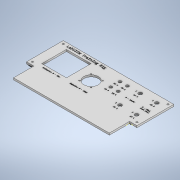
# Autodesk Inventor part: Labview Training Faceplate
Saved by Autodesk Inventor 2022 (Build 260153000, 153)
## iProperties
Created: 2022-07-29
Part Number: Labview Training Faceplate
Material: Generic
Document SubType Name: Modeling
Designer: dheard
Density: 1 g/cm^3
Appearance: Default
Author: dheard
Autodesk Inventor part; units mm, degrees
(part 1 of 3)
ref_plane "YZ Plane" through (0, 0, 0) normal (1, 0, 0) x (0, 1, 0)
ref_plane "XZ Plane" through (0, 0, 0) normal (0, 1, 0) x (-1, 0, 0)
ref_plane "XY Plane" through (0, 0, 0) normal (0, 0, 1) x (1, 0, 0)
sketch "Sketch1" plane through (0, 0, 0) normal (0, 1, 0) x (-1, 0, 0)
  line L0 (150, -50) -> (-150, -50)
  line L1 (-150, -50) -> (-150, 50)
  line L2 (150, 50) -> (150, -50)
  line L3 (-130, 50) -> (-130, 105)
  line L4 (-130, 105) -> (130, 105)
  line L5 (130, 105) -> (130, 50)
  line L6 (-150, 50) -> (-130, 50)
  line L7 (130, 50) -> (150, 50)
  point P0 (0, 0)
  dimension "d0" = 100
  dimension "d1" = 55
  dimension "d2" = 300
  dimension "d3" = 20
  dimension "d4" = 20
  dimension "d5" = 150
  dimension "d6" = 50
  constraints: 16 end point, 4 parallel, 2 horizontal alignment, 1 horizontal, 1 perpendicular
  measures "d0" distance between parallel lines of L7 L0
  measures "d1" distance between parallel lines of L4 L7
  measures "d2" distance between parallel lines of L1 L2
  measures "d3" distance between parallel lines of L5 L2
  measures "d4" distance between parallel lines of L1 L3
  measures "d5" distance from line of point (0, 0) L1
  measures "d6" distance from line of point (0, 0) L0
extrude "Extrusion1" add sketch "Sketch1" along normal blind 5
sketch "Sketch3" plane through (0, 5, 0) normal (0, 1, 0) x (1, 0, 0)
  line L0 (-125, 33.5) -> (-58, 33.5)
  line L1 (-58, 33.5) -> (-58, -33.5)
  line L2 (-58, -33.5) -> (-125, -33.5)
  line L3 (-125, -33.5) -> (-125, 33.5)
  line L4 (150, 50) -> (-150, 50) projected
  line L5 (-150, 50) -> (-150, -50) projected
  circle A0 centre (-18, -6.5) radius 19.5
  line L6 (-34, 9.5) -> (-2, 9.5) construction
  line L7 (-2, 9.5) -> (-2, -22.5) construction
  line L8 (-2, -22.5) -> (-34, -22.5) construction
  line L9 (-34, -22.5) -> (-34, 9.5) construction
  circle A1 centre (-34, 9.5) radius 1.5
  circle A2 centre (-2, -22.5) radius 1.5
  circle A3 centre (-34, -22.5) radius 1.5
  circle A4 centre (-2, 9.5) radius 1.5
  circle A5 centre (79, -25) radius 4.75
  circle A6 centre (79, 30) radius 4.75
  circle A7 centre (124, -25) radius 4.75
  circle A8 centre (124, 30) radius 4.75
  circle A9 centre (24, 5) radius 4
  circle A10 centre (44, 5) radius 4
  circle A11 centre (44, 30) radius 4
  circle A12 centre (24, 30) radius 4
  line L10 (68, 31.3) -> (68, 28.7) construction
  line L11 (68.65, 31.3) -> (68.65, 28.7)
  line L12 (67.35, 28.7) -> (67.35, 31.3)
  arc A13 (68.65, 31.3) -> (67.35, 31.3) centre (68, 31.3) ccw
  arc A14 (67.35, 28.7) -> (68.65, 28.7) centre (68, 28.7) ccw
  line L13 (68, -23.7) -> (68, -26.3) construction
  line L14 (68.65, -23.7) -> (68.65, -26.3)
  line L15 (67.35, -26.3) -> (67.35, -23.7)
  arc A15 (68.65, -23.7) -> (67.35, -23.7) centre (68, -23.7) ccw
  arc A16 (67.35, -26.3) -> (68.65, -26.3) centre (68, -26.3) ccw
  line L16 (112.35, -26.3) -> (112.35, -23.7)
  line L17 (113, -23.7) -> (113, -26.3) construction
  line L18 (113.65, -23.7) -> (113.65, -26.3)
  arc A17 (113.65, -23.7) -> (112.35, -23.7) centre (113, -23.7) ccw
  arc A18 (112.35, -26.3) -> (113.65, -26.3) centre (113, -26.3) ccw
  line L19 (112.35, 28.7) -> (112.35, 31.3)
  line L20 (113, 31.3) -> (113, 28.7) construction
  line L21 (113.65, 31.3) -> (113.65, 28.7)
  arc A19 (113.65, 31.3) -> (112.35, 31.3) centre (113, 31.3) ccw
  arc A20 (112.35, 28.7) -> (113.65, 28.7) centre (113, 28.7) ccw
  line L22 (-150, -50) -> (-130, -50) projected
  point P0 (68, 30)
  point P1 (68, -25)
  point P2 (113, -25)
  point P3 (113, 30)
  dimension "d11" = 67
  dimension "d12" = 67
  dimension "d13" = 16.5
  dimension "d15" = 25
  dimension "d16" = 39
  dimension "d17" = 40
  dimension "d18" = 40
  dimension "d19" = 32
  dimension "d20" = 32
  dimension "d23" = 16
  dimension "d24" = 16
  dimension "d25" = 3
  dimension "d26" = 3
  dimension "d27" = 3
  dimension "d28" = 3
  dimension "d29" = 9.5
  dimension "d30" = 45
  dimension "d31" = 55
  dimension "d32" = 20
  dimension "d34" = 8
  dimension "d36" = 20
  dimension "d37" = 25
  dimension "d38" = 20
  dimension "d39" = 42
  dimension "d40" = 35
  dimension "d41" = 11
  dimension "d42" = 2.6
  dimension "d43" = 1.3
  dimension "d44" = 2.6
  dimension "d45" = 1.3
  dimension "d46" = 2.6
  dimension "d47" = 1.3
  dimension "d48" = 2.6
  dimension "d49" = 1.3
  dimension "d50" = 11
  dimension "d65" = 16.5
  constraints: 48 end point, 21 centre point, 16 point on circle, 16 tangent, 8 horizontal alignment, 8 parallel, 6 equal radius, 6 vertical alignment, 4 coincident, 4 midpoint, 4 vertical, 2 horizontal, 2 perpendicular
  measures "d11" distance between parallel lines of L1 L3
  measures "d12" distance between parallel lines of L2 L0
  measures "d13" distance between parallel lines of L4 L0
  measures "d15" distance between parallel lines of L5 L3
  measures "d16" diameter of A0
  measures "d17" distance from line of L0 A0.centre
  measures "d18" distance from line of A0.centre L1
  measures "d19" distance between parallel lines of L7 L9
  measures "d20" distance between parallel lines of L6 L8
  measures "d23" distance from line of A0.centre L6
  measures "d24" distance from line of A0.centre L9
  measures "d25" diameter of A1
  measures "d26" diameter of A4
  measures "d27" diameter of A2
  measures "d28" diameter of A3
  measures "d29" diameter of A5
  measures "d30" distance of A8.centre A6.centre
  measures "d31" distance of A7.centre A8.centre
  measures "d32" distance from line of L4 A6.centre
  measures "d34" diameter of A9
  measures "d36" distance of A10.centre A9.centre
  measures "d37" distance of A10.centre A11.centre
  measures "d38" distance from line of L4 A12.centre
  measures "d39" horizontal distance of A0.centre A12.centre
  measures "d40" distance of A11.centre A6.centre
  measures "d41" distance of A6.centre point (68, 30)
  measures "d42" distance of L10.start L10.end
  measures "d43" distance between parallel lines of L11 L12
  measures "d44" distance of L13.start L13.end
  measures "d45" distance between parallel lines of L14 L15
  measures "d46" distance of L17.start L17.end
  measures "d47" distance between parallel lines of L18 L16
  measures "d48" distance of L20.start L20.end
  measures "d49" distance between parallel lines of L21 L19
  measures "d50" distance of A8.centre point (113, 30)
  measures "d65" distance between parallel lines of L22 L2
extrude "Extrusion2" cut sketch "Sketch3" against normal through all
sketch "Sketch4" plane through (0, 5, 0) normal (0, 1, 0) x (1, 0, 0)
  circle A0 centre (-142, 42) radius 2.25
  circle A1 centre (142, 42) radius 2.25
  circle A2 centre (-142, -42) radius 2.25
  circle A3 centre (142, -42) radius 2.25
  line L0 (-150, 50) -> (-150, -50) projected
  line L1 (150, 50) -> (-150, 50) projected
  line L2 (-150, -50) -> (-130, -50) projected
  line L3 (150, -50) -> (150, 50) projected
  point P0 (0, 0)
  dimension "d55" = 4.5
  dimension "d58" = 8
  dimension "d59" = 8
  dimension "d60" = 8
  dimension "d62" = 8
  constraints: 4 centre point, 3 equal radius, 2 horizontal alignment, 2 vertical alignment
  measures "d55" diameter of A0
  measures "d58" distance from line of L0 A0.centre
  measures "d59" distance from line of L1 A0.centre
  measures "d60" distance from line of L2 A2.centre
  measures "d62" distance from line of L3 A1.centre
extrude "Extrusion3" cut sketch "Sketch4" against normal blind 10
sketch "Sketch5" plane through (0, 5, 0) normal (0, 1, 0) x (1, 0, 0)
  line L0 (-131.9692, 46) -> (-24.524, 46) construction
  line L1 (-24.524, 46) -> (-24.524, 37.1257) construction
  line L2 (-24.524, 37.1257) -> (-131.9692, 37.1257) construction
  line L3 (-131.9692, 37.1257) -> (-131.9692, 46) construction
  line L4 (-115, -39) -> (-68, -39) construction
  line L5 (-68, -39) -> (-68, -43.7381) construction
  line L6 (-68, -43.7381) -> (-115, -43.7381) construction
  line L7 (-115, -43.7381) -> (-115, -39) construction
  line L8 (-41, -43.9686) -> (-41, -39) construction
  line L9 (-41, -39) -> (5, -39) construction
  line L10 (5, -39) -> (5, -43.9686) construction
  line L11 (5, -43.9686) -> (-41, -43.9686) construction
  line L12 (19, 14.2768) -> (19, 20) construction
  line L13 (19, 20) -> (30.6254, 20) construction
  line L14 (30.6254, 20) -> (30.6254, 14.2768) construction
  line L15 (30.6254, 14.2768) -> (19, 14.2768) construction
  line L16 (39, 14.2768) -> (39, 20) construction
  line L17 (39, 20) -> (50.0529, 20) construction
  line L18 (50.0529, 20) -> (50.0529, 14.2768) construction
  line L19 (50.0529, 14.2768) -> (39, 14.2768) construction
  line L20 (19, -10.7232) -> (19, -5) construction
  line L21 (19, -5) -> (31.5796, -5) construction
  line L22 (31.5796, -5) -> (31.5796, -10.7232) construction
  line L23 (31.5796, -10.7232) -> (19, -10.7232) construction
  line L24 (39, -10.7232) -> (39, -5) construction
  line L25 (39, -5) -> (50.0917, -5) construction
  line L26 (50.0917, -5) -> (50.0917, -10.7232) construction
  line L27 (50.0917, -10.7232) -> (39, -10.7232) construction
  line L28 (68, -2.5818) -> (68, 3) construction
  line L29 (68, 3) -> (94.3213, 3) construction
  line L30 (94.3213, 3) -> (94.3213, -2.5818) construction
  line L31 (94.3213, -2.5818) -> (68, -2.5818) construction
  line L32 (113, -2.5818) -> (113, 3) construction
  line L33 (113, 3) -> (139.3213, 3) construction
  line L34 (139.3213, 3) -> (139.3213, -2.5818) construction
  line L35 (139.3213, -2.5818) -> (113, -2.5818) construction
  line L36 (113, -6.8453) -> (113, -2.353) construction
  line L37 (113, -2.353) -> (137.7599, -2.353) construction
  line L38 (137.7599, -2.353) -> (137.7599, -6.8453) construction
  line L39 (137.7599, -6.8453) -> (113, -6.8453) construction
  line L40 (73, 14.4182) -> (73, 20) construction
  line L41 (73, 20) -> (86.5493, 20) construction
  line L42 (86.5493, 20) -> (86.5493, 14.4182) construction
  line L43 (86.5493, 14.4182) -> (73, 14.4182) construction
  line L44 (73, -40.5818) -> (73, -35) construction
  line L45 (73, -35) -> (86.5493, -35) construction
  line L46 (86.5493, -35) -> (86.5493, -40.5818) construction
  line L47 (86.5493, -40.5818) -> (73, -40.5818) construction
  line L48 (118, 14.4182) -> (118, 20) construction
  line L49 (118, 20) -> (131.5493, 20) construction
  line L50 (131.5493, 20) -> (131.5493, 14.4182) construction
  line L51 (131.5493, 14.4182) -> (118, 14.4182) construction
  line L52 (118, -40.5818) -> (118, -35) construction
  line L53 (118, -35) -> (131.5493, -35) construction
  line L54 (131.5493, -35) -> (131.5493, -40.5818) construction
  line L55 (131.5493, -40.5818) -> (118, -40.5818) construction
  circle A0 centre (24, 30) radius 4 projected
  circle A1 centre (24, 5) radius 4 projected
  circle A2 centre (44, 30) radius 4 projected
  circle A3 centre (79, 30) radius 4.75 projected
  circle A4 centre (124, 30) radius 4.75 projected
  circle A5 centre (79, -25) radius 4.75 projected
  line L56 (-150, -50) -> (-130, -50) projected
  line L57 (-125, -33.5) -> (-125, 33.5) projected
  line L58 (-58, 33.5) -> (-58, -33.5) projected
  circle A6 centre (-18, -6.5) radius 19.5 projected
  line L59 (150, 50) -> (-150, 50) projected
  line L60 (-127.3724, 39.3479) -> (-130.8815, 39.3479)
  line L61 (-130.8815, 39.3479) -> (-130.8815, 45.4479)
  line L62 (-130.8815, 45.4479) -> (-130.0343, 45.4479)
  line L63 (-130.0343, 45.4479) -> (-130.0343, 40.0585)
  line L64 (-130.0343, 40.0585) -> (-127.3724, 40.0585)
  line L65 (-127.3724, 40.0585) -> (-127.3724, 39.3479)
  line L66 (-122.9504, 39.3479) -> (-122.9668, 39.9765)
  spline S0 degree 2 poles (-122.9668, 39.9765) (-123.3494, 39.5994) (-124.142, 39.2659) (-124.5738, 39.2659) knots 0 0 0 1 2 2 2
  spline S1 degree 2 poles (-124.5738, 39.2659) (-124.9783, 39.2659) (-125.5467, 39.4737) (-125.913, 39.8289) (-126.0879, 40.3154) (-126.0879, 40.5996) knots 0 0 0 1 2 3 4 4 4
  spline S2 degree 2 poles (-126.0879, 40.5996) (-126.0879, 41.3047) (-125.0384, 42.1028) (-124.0108, 42.1028) knots 0 0 0 1 2 2 2
  line L67 (-124.0108, 42.1028) -> (-123.0379, 42.1028)
  line L68 (-123.0379, 42.1028) -> (-123.0379, 42.5127)
  spline S3 degree 2 poles (-123.0379, 42.5127) (-123.0379, 42.9281) (-123.5681, 43.431) (-124.1147, 43.431) knots 0 0 0 1 2 2 2
  spline S4 degree 2 poles (-124.1147, 43.431) (-124.5137, 43.431) (-125.2844, 43.2561) (-125.6943, 43.0921) knots 0 0 0 1 2 2 2
  line L69 (-125.6943, 43.0921) -> (-125.6943, 43.8246)
  spline S5 degree 2 poles (-125.6943, 43.8246) (-125.5413, 43.8792) (-125.1641, 43.9885) (-124.7433, 44.0705) (-124.2841, 44.1197) (-124.0545, 44.1197) knots 0 0 0 1 2 3 4 4 4
  spline S6 degree 2 poles (-124.0545, 44.1197) (-123.6282, 44.1197) (-122.945, 43.9339) (-122.4749, 43.5513) (-122.2234, 42.9719) (-122.2234, 42.5783) knots 0 0 0 1 2 3 4 4 4
  line L70 (-122.2234, 42.5783) -> (-122.2234, 39.3479)
  line L71 (-122.2234, 39.3479) -> (-122.9504, 39.3479)
  line L72 (-123.0379, 41.4797) -> (-124.0709, 41.4797)
  spline S7 degree 2 poles (-124.0709, 41.4797) (-124.377, 41.4797) (-124.8143, 41.3594) (-125.0931, 41.1353) (-125.2297, 40.8237) (-125.2297, 40.627) knots 0 0 0 1 2 3 4 4 4
  spline S8 degree 2 poles (-125.2297, 40.627) (-125.2297, 40.4903) (-125.1477, 40.2444) (-124.9564, 40.053) (-124.6613, 39.9437) (-124.4426, 39.9437) knots 0 0 0 1 2 3 4 4 4
  spline S9 degree 2 poles (-124.4426, 39.9437) (-124.1639, 39.9437) (-123.4424, 40.2826) (-123.0379, 40.6488) knots 0 0 0 1 2 2 2
  line L73 (-123.0379, 40.6488) -> (-123.0379, 41.4797)
  spline S10 degree 2 poles (-116.6974, 41.7748) (-116.6974, 41.1954) (-117.0199, 40.2717) (-117.6102, 39.6322) (-118.4629, 39.2933) (-118.9931, 39.2933) knots 0 0 0 1 2 3 4 4 4
  spline S11 degree 2 poles (-118.9931, 39.2933) (-119.4085, 39.2933) (-120.2776, 39.4518) (-120.7039, 39.6267) knots 0 0 0 1 2 2 2
  line L74 (-120.7039, 39.6267) -> (-120.7039, 45.9453)
  line L75 (-120.7039, 45.9453) -> (-119.8895, 45.9453)
  line L76 (-119.8895, 45.9453) -> (-119.8895, 44.1306)
  line L77 (-119.8895, 44.1306) -> (-119.9277, 43.2616)
  spline S12 degree 2 poles (-119.9277, 43.2616) (-119.5779, 43.7316) (-118.7799, 44.1197) (-118.3208, 44.1197) knots 0 0 0 1 2 2 2
  spline S13 degree 2 poles (-118.3208, 44.1197) (-117.9217, 44.1197) (-117.315, 43.7863) (-116.9051, 43.1741) (-116.6974, 42.3105) (-116.6974, 41.7748) knots 0 0 0 1 2 3 4 4 4
  spline S14 degree 2 poles (-117.5282, 41.7366) (-117.5282, 42.1082) (-117.6375, 42.7204) (-117.8671, 43.1632) (-118.2333, 43.4091) (-118.4847, 43.4091) knots 0 0 0 1 2 3 4 4 4
  spline S15 degree 2 poles (-118.4847, 43.4091) (-118.6378, 43.4091) (-118.9548, 43.3108) (-119.2992, 43.0812) (-119.6763, 42.704) (-119.8895, 42.4253) knots 0 0 0 1 2 3 4 4 4
  line L78 (-119.8895, 42.4253) -> (-119.8895, 40.1514)
  spline S16 degree 2 poles (-119.8895, 40.1514) (-119.649, 40.0585) (-119.1571, 39.9492) (-118.9329, 39.9492) knots 0 0 0 1 2 2 2
  spline S17 degree 2 poles (-118.9329, 39.9492) (-118.6542, 39.9492) (-118.1458, 40.1241) (-117.7578, 40.5395) (-117.5282, 41.2282) (-117.5282, 41.7366) knots 0 0 0 1 2 3 4 4 4
  line L79 (-110.9527, 45.4479) -> (-113.0297, 39.3479)
  line L80 (-113.0297, 39.3479) -> (-114.1502, 39.3479)
  line L81 (-114.1502, 39.3479) -> (-116.1726, 45.4479)
  line L82 (-116.1726, 45.4479) -> (-115.238, 45.4479)
  line L83 (-115.238, 45.4479) -> (-113.9207, 41.3375)
  line L84 (-113.9207, 41.3375) -> (-113.5435, 40.1296)
  line L85 (-113.5435, 40.1296) -> (-113.1609, 41.3375)
  line L86 (-113.1609, 41.3375) -> (-111.8436, 45.4479)
  line L87 (-111.8436, 45.4479) -> (-110.9527, 45.4479)
  line L88 (-108.728, 44.7483) -> (-110.1328, 44.7483)
  line L89 (-110.1328, 44.7483) -> (-110.1328, 45.4479)
  line L90 (-110.1328, 45.4479) -> (-106.4815, 45.4479)
  line L91 (-106.4815, 45.4479) -> (-106.4815, 44.7483)
  line L92 (-106.4815, 44.7483) -> (-107.8863, 44.7483)
  line L93 (-107.8863, 44.7483) -> (-107.8863, 40.0585)
  line L94 (-107.8863, 40.0585) -> (-106.4815, 40.0585)
  line L95 (-106.4815, 40.0585) -> (-106.4815, 39.3479)
  line L96 (-106.4815, 39.3479) -> (-110.1328, 39.3479)
  line L97 (-110.1328, 39.3479) -> (-110.1328, 40.0585)
  line L98 (-110.1328, 40.0585) -> (-108.728, 40.0585)
  line L99 (-108.728, 40.0585) -> (-108.728, 44.7483)
  line L100 (-101.267, 39.3479) -> (-104.7379, 39.3479)
  line L101 (-104.7379, 39.3479) -> (-104.7379, 45.4479)
  line L102 (-104.7379, 45.4479) -> (-101.267, 45.4479)
  line L103 (-101.267, 45.4479) -> (-101.267, 44.7483)
  line L104 (-101.267, 44.7483) -> (-103.9071, 44.7483)
  line L105 (-103.9071, 44.7483) -> (-103.9071, 42.8571)
  line L106 (-103.9071, 42.8571) -> (-101.3708, 42.8571)
  line L107 (-101.3708, 42.8571) -> (-101.3708, 42.1574)
  line L108 (-101.3708, 42.1574) -> (-103.9071, 42.1574)
  line L109 (-103.9071, 42.1574) -> (-103.9071, 40.0585)
  line L110 (-103.9071, 40.0585) -> (-101.267, 40.0585)
  line L111 (-101.267, 40.0585) -> (-101.267, 39.3479)
  line L112 (-95.3747, 45.4479) -> (-95.7846, 39.3479)
  line L113 (-95.7846, 39.3479) -> (-96.8614, 39.3479)
  line L114 (-96.8614, 39.3479) -> (-97.6212, 41.5179)
  line L115 (-97.6212, 41.5179) -> (-97.8289, 42.2121)
  line L116 (-97.8289, 42.2121) -> (-98.0476, 41.4633)
  line L117 (-98.0476, 41.4633) -> (-98.7527, 39.3479)
  line L118 (-98.7527, 39.3479) -> (-99.7912, 39.3479)
  line L119 (-99.7912, 39.3479) -> (-100.2121, 45.4479)
  line L120 (-100.2121, 45.4479) -> (-99.4304, 45.4479)
  line L121 (-99.4304, 45.4479) -> (-99.1899, 41.2938)
  line L122 (-99.1899, 41.2938) -> (-99.1189, 40.1569)
  line L123 (-99.1189, 40.1569) -> (-98.8237, 41.1244)
  line L124 (-98.8237, 41.1244) -> (-98.0858, 43.3873)
  line L125 (-98.0858, 43.3873) -> (-97.5119, 43.3873)
  line L126 (-97.5119, 43.3873) -> (-96.6592, 40.9604)
  line L127 (-96.6592, 40.9604) -> (-96.375, 40.1569)
  line L128 (-96.375, 40.1569) -> (-96.3586, 40.9932)
  line L129 (-96.3586, 40.9932) -> (-96.1181, 45.4479)
  line L130 (-96.1181, 45.4479) -> (-95.3747, 45.4479)
  line L131 (-85.0441, 44.7374) -> (-86.8533, 44.7374)
  line L132 (-86.8533, 44.7374) -> (-86.8533, 39.3479)
  line L133 (-86.8533, 39.3479) -> (-87.695, 39.3479)
  line L134 (-87.695, 39.3479) -> (-87.695, 44.7374)
  line L135 (-87.695, 44.7374) -> (-89.5043, 44.7374)
  line L136 (-89.5043, 44.7374) -> (-89.5043, 45.4479)
  line L137 (-89.5043, 45.4479) -> (-85.0441, 45.4479)
  line L138 (-85.0441, 45.4479) -> (-85.0441, 44.7374)
  line L139 (-83.7049, 44.0323) -> (-82.9615, 44.0323)
  line L140 (-82.9615, 44.0323) -> (-82.9397, 43.1686)
  spline S18 degree 2 poles (-82.9397, 43.1686) (-82.5243, 43.6715) (-81.7208, 44.1197) (-81.3053, 44.1197) knots 0 0 0 1 2 2 2
  spline S19 degree 2 poles (-81.3053, 44.1197) (-80.5784, 44.1197) (-79.8295, 43.1741) (-79.8569, 42.2449) knots 0 0 0 1 2 2 2
  line L141 (-79.8569, 42.2449) -> (-80.6768, 42.2449)
  spline S20 degree 2 poles (-80.6768, 42.2449) (-80.6604, 42.8625) (-81.0484, 43.4201) (-81.4256, 43.4201) knots 0 0 0 1 2 2 2
  spline S21 degree 2 poles (-81.4256, 43.4201) (-81.5896, 43.4201) (-81.9175, 43.3053) (-82.2674, 43.0429) (-82.6609, 42.6439) (-82.885, 42.3542) knots 0 0 0 1 2 3 4 4 4
  line L142 (-82.885, 42.3542) -> (-82.885, 39.3479)
  line L143 (-82.885, 39.3479) -> (-83.7049, 39.3479)
  line L144 (-83.7049, 39.3479) -> (-83.7049, 44.0323)
  line L145 (-75.6262, 39.3479) -> (-75.6426, 39.9765)
  spline S22 degree 2 poles (-75.6426, 39.9765) (-76.0252, 39.5994) (-76.8178, 39.2659) (-77.2496, 39.2659) knots 0 0 0 1 2 2 2
  spline S23 degree 2 poles (-77.2496, 39.2659) (-77.6541, 39.2659) (-78.2226, 39.4737) (-78.5888, 39.8289) (-78.7637, 40.3154) (-78.7637, 40.5996) knots 0 0 0 1 2 3 4 4 4
  spline S24 degree 2 poles (-78.7637, 40.5996) (-78.7637, 41.3047) (-77.7142, 42.1028) (-76.6866, 42.1028) knots 0 0 0 1 2 2 2
  line L146 (-76.6866, 42.1028) -> (-75.7137, 42.1028)
  line L147 (-75.7137, 42.1028) -> (-75.7137, 42.5127)
  spline S25 degree 2 poles (-75.7137, 42.5127) (-75.7137, 42.9281) (-76.2439, 43.431) (-76.7905, 43.431) knots 0 0 0 1 2 2 2
  spline S26 degree 2 poles (-76.7905, 43.431) (-77.1895, 43.431) (-77.9602, 43.2561) (-78.3701, 43.0921) knots 0 0 0 1 2 2 2
  line L148 (-78.3701, 43.0921) -> (-78.3701, 43.8246)
  spline S27 degree 2 poles (-78.3701, 43.8246) (-78.2171, 43.8792) (-77.8399, 43.9885) (-77.4191, 44.0705) (-76.9599, 44.1197) (-76.7303, 44.1197) knots 0 0 0 1 2 3 4 4 4
  spline S28 degree 2 poles (-76.7303, 44.1197) (-76.304, 44.1197) (-75.6208, 43.9339) (-75.1507, 43.5513) (-74.8993, 42.9719) (-74.8993, 42.5783) knots 0 0 0 1 2 3 4 4 4
  line L149 (-74.8993, 42.5783) -> (-74.8993, 39.3479)
  line L150 (-74.8993, 39.3479) -> (-75.6262, 39.3479)
  line L151 (-75.7137, 41.4797) -> (-76.7467, 41.4797)
  spline S29 degree 2 poles (-76.7467, 41.4797) (-77.0528, 41.4797) (-77.4901, 41.3594) (-77.7689, 41.1353) (-77.9055, 40.8237) (-77.9055, 40.627) knots 0 0 0 1 2 3 4 4 4
  spline S30 degree 2 poles (-77.9055, 40.627) (-77.9055, 40.4903) (-77.8235, 40.2444) (-77.6322, 40.053) (-77.3371, 39.9437) (-77.1184, 39.9437) knots 0 0 0 1 2 3 4 4 4
  spline S31 degree 2 poles (-77.1184, 39.9437) (-76.8397, 39.9437) (-76.1182, 40.2826) (-75.7137, 40.6488) knots 0 0 0 1 2 2 2
  line L152 (-75.7137, 40.6488) -> (-75.7137, 41.4797)
  line L153 (-71.7837, 43.3599) -> (-73.172, 43.3599)
  line L154 (-73.172, 43.3599) -> (-73.172, 44.0323)
  line L155 (-73.172, 44.0323) -> (-70.9638, 44.0323)
  line L156 (-70.9638, 44.0323) -> (-70.9638, 40.0257)
  line L157 (-70.9638, 40.0257) -> (-69.57, 40.0257)
  line L158 (-69.57, 40.0257) -> (-69.57, 39.3479)
  line L159 (-69.57, 39.3479) -> (-73.3251, 39.3479)
  line L160 (-73.3251, 39.3479) -> (-73.3251, 40.0257)
  line L161 (-73.3251, 40.0257) -> (-71.7837, 40.0257)
  line L162 (-71.7837, 40.0257) -> (-71.7837, 43.3599)
  spline S32 degree 2 poles (-71.4994, 46) (-71.3628, 46) (-71.1332, 45.9016) (-70.9583, 45.7267) (-70.8599, 45.4971) (-70.8599, 45.3605) knots 0 0 0 1 2 3 4 4 4
  spline S33 degree 2 poles (-70.8599, 45.3605) (-70.8599, 45.2293) (-70.9583, 44.9943) (-71.1332, 44.8194) (-71.3628, 44.721) (-71.4994, 44.721) knots 0 0 0 1 2 3 4 4 4
  spline S34 degree 2 poles (-71.4994, 44.721) (-71.6361, 44.721) (-71.8657, 44.8194) (-72.0406, 44.9943) (-72.1389, 45.2293) (-72.1389, 45.3605) knots 0 0 0 1 2 3 4 4 4
  spline S35 degree 2 poles (-72.1389, 45.3605) (-72.1389, 45.4971) (-72.0406, 45.7267) (-71.8657, 45.9016) (-71.6361, 46) (-71.4994, 46) knots 0 0 0 1 2 3 4 4 4
  line L163 (-68.1215, 44.0323) -> (-67.3945, 44.0323)
  line L164 (-67.3945, 44.0323) -> (-67.3617, 43.278)
  spline S36 degree 2 poles (-67.3617, 43.278) (-67.1595, 43.5185) (-66.7769, 43.8409) (-66.4052, 44.0377) (-66.0226, 44.1197) (-65.8148, 44.1197) knots 0 0 0 1 2 3 4 4 4
  spline S37 degree 2 poles (-65.8148, 44.1197) (-65.0933, 44.1197) (-64.35, 43.267) (-64.35, 42.4089) knots 0 0 0 1 2 2 2
  line L165 (-64.35, 42.4089) -> (-64.35, 39.3479)
  line L166 (-64.35, 39.3479) -> (-65.1644, 39.3479)
  line L167 (-65.1644, 39.3479) -> (-65.1644, 42.3433)
  spline S38 degree 2 poles (-65.1644, 42.3433) (-65.1644, 42.8899) (-65.5743, 43.4201) (-65.9788, 43.4201) knots 0 0 0 1 2 2 2
  spline S39 degree 2 poles (-65.9788, 43.4201) (-66.1319, 43.4201) (-66.4161, 43.3326) (-66.7222, 43.114) (-67.0829, 42.7368) (-67.307, 42.4581) knots 0 0 0 1 2 3 4 4 4
  line L168 (-67.307, 42.4581) -> (-67.307, 39.3479)
  line L169 (-67.307, 39.3479) -> (-68.1215, 39.3479)
  line L170 (-68.1215, 39.3479) -> (-68.1215, 44.0323)
  line L171 (-61.2672, 43.3599) -> (-62.6555, 43.3599)
  line L172 (-62.6555, 43.3599) -> (-62.6555, 44.0323)
  line L173 (-62.6555, 44.0323) -> (-60.4473, 44.0323)
  line L174 (-60.4473, 44.0323) -> (-60.4473, 40.0257)
  line L175 (-60.4473, 40.0257) -> (-59.0535, 40.0257)
  line L176 (-59.0535, 40.0257) -> (-59.0535, 39.3479)
  line L177 (-59.0535, 39.3479) -> (-62.8086, 39.3479)
  line L178 (-62.8086, 39.3479) -> (-62.8086, 40.0257)
  line L179 (-62.8086, 40.0257) -> (-61.2672, 40.0257)
  line L180 (-61.2672, 40.0257) -> (-61.2672, 43.3599)
  spline S40 degree 2 poles (-60.9829, 46) (-60.8463, 46) (-60.6167, 45.9016) (-60.4418, 45.7267) (-60.3434, 45.4971) (-60.3434, 45.3605) knots 0 0 0 1 2 3 4 4 4
  spline S41 degree 2 poles (-60.3434, 45.3605) (-60.3434, 45.2293) (-60.4418, 44.9943) (-60.6167, 44.8194) (-60.8463, 44.721) (-60.9829, 44.721) knots 0 0 0 1 2 3 4 4 4
  spline S42 degree 2 poles (-60.9829, 44.721) (-61.1196, 44.721) (-61.3492, 44.8194) (-61.5241, 44.9943) (-61.6225, 45.2293) (-61.6225, 45.3605) knots 0 0 0 1 2 3 4 4 4
  spline S43 degree 2 poles (-61.6225, 45.3605) (-61.6225, 45.4971) (-61.5241, 45.7267) (-61.3492, 45.9016) (-61.1196, 46) (-60.9829, 46) knots 0 0 0 1 2 3 4 4 4
  line L181 (-57.605, 44.0323) -> (-56.878, 44.0323)
  line L182 (-56.878, 44.0323) -> (-56.8452, 43.278)
  spline S44 degree 2 poles (-56.8452, 43.278) (-56.643, 43.5185) (-56.2604, 43.8409) (-55.8887, 44.0377) (-55.5061, 44.1197) (-55.2984, 44.1197) knots 0 0 0 1 2 3 4 4 4
  spline S45 degree 2 poles (-55.2984, 44.1197) (-54.5769, 44.1197) (-53.8335, 43.267) (-53.8335, 42.4089) knots 0 0 0 1 2 2 2
  line L183 (-53.8335, 42.4089) -> (-53.8335, 39.3479)
  line L184 (-53.8335, 39.3479) -> (-54.6479, 39.3479)
  line L185 (-54.6479, 39.3479) -> (-54.6479, 42.3433)
  spline S46 degree 2 poles (-54.6479, 42.3433) (-54.6479, 42.8899) (-55.0579, 43.4201) (-55.4623, 43.4201) knots 0 0 0 1 2 2 2
  spline S47 degree 2 poles (-55.4623, 43.4201) (-55.6154, 43.4201) (-55.8996, 43.3326) (-56.2057, 43.114) (-56.5665, 42.7368) (-56.7906, 42.4581) knots 0 0 0 1 2 3 4 4 4
  line L186 (-56.7906, 42.4581) -> (-56.7906, 39.3479)
  line L187 (-56.7906, 39.3479) -> (-57.605, 39.3479)
  line L188 (-57.605, 39.3479) -> (-57.605, 44.0323)
  spline S48 degree 2 poles (-48.9743, 43.3709) (-48.8431, 43.2069) (-48.701, 42.7751) (-48.701, 42.5237) knots 0 0 0 1 2 2 2
  spline S49 degree 2 poles (-48.701, 42.5237) (-48.701, 42.1574) (-48.9688, 41.5562) (-49.4498, 41.1298) (-50.1276, 40.8893) (-50.532, 40.8893) knots 0 0 0 1 2 3 4 4 4
  spline S50 degree 2 poles (-50.532, 40.8893) (-50.8272, 40.8893) (-51.341, 41.0151) (-51.4886, 41.108) knots 0 0 0 1 2 2 2
  spline S51 degree 2 poles (-51.4886, 41.108) (-51.5815, 40.9768) (-51.7018, 40.7472) (-51.7018, 40.5996) knots 0 0 0 1 2 2 2
  spline S52 degree 2 poles (-51.7018, 40.5996) (-51.7018, 40.4247) (-51.3629, 40.1897) (-51.0786, 40.1788) knots 0 0 0 1 2 2 2
  line L189 (-51.0786, 40.1788) -> (-49.8488, 40.135)
  spline S53 degree 2 poles (-49.8488, 40.135) (-49.499, 40.1241) (-48.9032, 39.9656) (-48.4823, 39.665) (-48.2418, 39.2277) (-48.2418, 38.938) knots 0 0 0 1 2 3 4 4 4
  spline S54 degree 2 poles (-48.2418, 38.938) (-48.2418, 38.6264) (-48.5151, 38.0634) (-49.0781, 37.6371) (-49.9472, 37.3857) (-50.543, 37.3857) knots 0 0 0 1 2 3 4 4 4
  spline S55 degree 2 poles (-50.543, 37.3857) (-51.1114, 37.3857) (-51.9095, 37.566) (-52.4233, 37.8885) (-52.6583, 38.3313) (-52.6583, 38.5991) knots 0 0 0 1 2 3 4 4 4
  spline S56 degree 2 poles (-52.6583, 38.5991) (-52.6583, 38.9435) (-52.3413, 39.4573) (-52.0079, 39.6923) knots 0 0 0 1 2 2 2
  spline S57 degree 2 poles (-52.0079, 39.6923) (-52.1336, 39.747) (-52.3085, 39.9164) (-52.4233, 40.1186) (-52.4779, 40.3427) (-52.4779, 40.4521) knots 0 0 0 1 2 3 4 4 4
  spline S58 degree 2 poles (-52.4779, 40.4521) (-52.4779, 40.7527) (-52.1937, 41.2556) (-51.9969, 41.4797) knots 0 0 0 1 2 2 2
  spline S59 degree 2 poles (-51.9969, 41.4797) (-52.0844, 41.589) (-52.221, 41.7967) (-52.3194, 42.0317) (-52.3686, 42.3105) (-52.3686, 42.4854) knots 0 0 0 1 2 3 4 4 4
  spline S60 degree 2 poles (-52.3686, 42.4854) (-52.3686, 42.8516) (-52.1008, 43.4529) (-51.6198, 43.8792) (-50.9475, 44.1197) (-50.5375, 44.1197) knots 0 0 0 1 2 3 4 4 4
  spline S61 degree 2 poles (-50.5375, 44.1197) (-50.3626, 44.1197) (-50.0456, 44.0705) (-49.9253, 44.0323) knots 0 0 0 1 2 2 2
  line L190 (-49.9253, 44.0323) -> (-48.2254, 44.0323)
  line L191 (-48.2254, 44.0323) -> (-48.2254, 43.3709)
  line L192 (-48.2254, 43.3709) -> (-48.9743, 43.3709)
  spline S62 degree 2 poles (-51.5487, 42.5073) (-51.5487, 42.2832) (-51.4011, 41.906) (-51.1278, 41.6436) (-50.7616, 41.5015) (-50.532, 41.5015) knots 0 0 0 1 2 3 4 4 4
  spline S63 degree 2 poles (-50.532, 41.5015) (-50.2915, 41.5015) (-49.9144, 41.6655) (-49.6575, 41.9443) (-49.5208, 42.3105) (-49.5208, 42.5073) knots 0 0 0 1 2 3 4 4 4
  spline S64 degree 2 poles (-49.5208, 42.5073) (-49.5208, 42.7259) (-49.6684, 43.103) (-49.9417, 43.3654) (-50.3079, 43.5075) (-50.532, 43.5075) knots 0 0 0 1 2 3 4 4 4
  spline S65 degree 2 poles (-50.532, 43.5075) (-50.778, 43.5075) (-51.1552, 43.3381) (-51.4121, 43.0648) (-51.5487, 42.6986) (-51.5487, 42.5073) knots 0 0 0 1 2 3 4 4 4
  spline S66 degree 2 poles (-51.7947, 38.6702) (-51.7947, 38.3422) (-51.106, 38.0361) (-50.4883, 38.0361) knots 0 0 0 1 2 2 2
  spline S67 degree 2 poles (-50.4883, 38.0361) (-50.1002, 38.0361) (-49.5755, 38.1782) (-49.253, 38.4023) (-49.1109, 38.6975) (-49.1109, 38.8505) knots 0 0 0 1 2 3 4 4 4
  spline S68 degree 2 poles (-49.1109, 38.8505) (-49.1109, 39.1348) (-49.5755, 39.4081) (-50.0565, 39.4299) knots 0 0 0 1 2 2 2
  line L193 (-50.0565, 39.4299) -> (-51.2809, 39.4737)
  spline S69 degree 2 poles (-51.2809, 39.4737) (-51.4339, 39.3698) (-51.6362, 39.173) (-51.7455, 38.9763) (-51.7947, 38.774) (-51.7947, 38.6702) knots 0 0 0 1 2 3 4 4 4
  line L194 (-37.6707, 39.3479) -> (-38.6108, 39.3479)
  line L195 (-38.6108, 39.3479) -> (-39.5236, 41.2993)
  spline S70 degree 2 poles (-39.5236, 41.2993) (-39.622, 41.5234) (-39.8407, 41.8185) (-40.0866, 41.988) (-40.3818, 42.0645) (-40.5622, 42.0645) knots 0 0 0 1 2 3 4 4 4
  line L196 (-40.5622, 42.0645) -> (-40.9557, 42.0645)
  line L197 (-40.9557, 42.0645) -> (-40.9557, 39.3479)
  line L198 (-40.9557, 39.3479) -> (-41.7865, 39.3479)
  line L199 (-41.7865, 39.3479) -> (-41.7865, 45.4479)
  line L200 (-41.7865, 45.4479) -> (-40.1522, 45.4479)
  spline S71 degree 2 poles (-40.1522, 45.4479) (-39.622, 45.4479) (-38.8568, 45.2129) (-38.3648, 44.792) (-38.1353, 44.2017) (-38.1353, 43.8409) knots 0 0 0 1 2 3 4 4 4
  spline S72 degree 2 poles (-38.1353, 43.8409) (-38.1353, 43.5567) (-38.3047, 43.0484) (-38.6327, 42.633) (-39.1246, 42.3323) (-39.4416, 42.2558) knots 0 0 0 1 2 3 4 4 4
  spline S73 degree 2 poles (-39.4416, 42.2558) (-39.1847, 42.1684) (-38.824, 41.7256) (-38.6381, 41.3539) knots 0 0 0 1 2 2 2
  line L201 (-38.6381, 41.3539) -> (-37.6707, 39.3479)
  spline S74 degree 2 poles (-39.0044, 43.7699) (-39.0044, 44.2618) (-39.6165, 44.7483) (-40.1741, 44.7483) knots 0 0 0 1 2 2 2
  line L202 (-40.1741, 44.7483) -> (-40.9557, 44.7483)
  line L203 (-40.9557, 44.7483) -> (-40.9557, 42.7314)
  line L204 (-40.9557, 42.7314) -> (-40.2834, 42.7314)
  spline S75 degree 2 poles (-40.2834, 42.7314) (-39.9882, 42.7314) (-39.5182, 42.868) (-39.1847, 43.1304) (-39.0044, 43.5185) (-39.0044, 43.7699) knots 0 0 0 1 2 3 4 4 4
  line L205 (-34.976, 43.3599) -> (-36.3643, 43.3599)
  line L206 (-36.3643, 43.3599) -> (-36.3643, 44.0323)
  line L207 (-36.3643, 44.0323) -> (-34.1561, 44.0323)
  line L208 (-34.1561, 44.0323) -> (-34.1561, 40.0257)
  line L209 (-34.1561, 40.0257) -> (-32.7622, 40.0257)
  line L210 (-32.7622, 40.0257) -> (-32.7622, 39.3479)
  line L211 (-32.7622, 39.3479) -> (-36.5174, 39.3479)
  line L212 (-36.5174, 39.3479) -> (-36.5174, 40.0257)
  line L213 (-36.5174, 40.0257) -> (-34.976, 40.0257)
  line L214 (-34.976, 40.0257) -> (-34.976, 43.3599)
  spline S76 degree 2 poles (-34.6917, 46) (-34.5551, 46) (-34.3255, 45.9016) (-34.1506, 45.7267) (-34.0522, 45.4971) (-34.0522, 45.3605) knots 0 0 0 1 2 3 4 4 4
  spline S77 degree 2 poles (-34.0522, 45.3605) (-34.0522, 45.2293) (-34.1506, 44.9943) (-34.3255, 44.8194) (-34.5551, 44.721) (-34.6917, 44.721) knots 0 0 0 1 2 3 4 4 4
  spline S78 degree 2 poles (-34.6917, 44.721) (-34.8284, 44.721) (-35.0579, 44.8194) (-35.2329, 44.9943) (-35.3312, 45.2293) (-35.3312, 45.3605) knots 0 0 0 1 2 3 4 4 4
  spline S79 degree 2 poles (-35.3312, 45.3605) (-35.3312, 45.4971) (-35.2329, 45.7267) (-35.0579, 45.9016) (-34.8284, 46) (-34.6917, 46) knots 0 0 0 1 2 3 4 4 4
  spline S80 degree 2 poles (-27.9413, 43.3709) (-27.8101, 43.2069) (-27.668, 42.7751) (-27.668, 42.5237) knots 0 0 0 1 2 2 2
  spline S81 degree 2 poles (-27.668, 42.5237) (-27.668, 42.1574) (-27.9358, 41.5562) (-28.4168, 41.1298) (-29.0946, 40.8893) (-29.4991, 40.8893) knots 0 0 0 1 2 3 4 4 4
  spline S82 degree 2 poles (-29.4991, 40.8893) (-29.7942, 40.8893) (-30.308, 41.0151) (-30.4556, 41.108) knots 0 0 0 1 2 2 2
  spline S83 degree 2 poles (-30.4556, 41.108) (-30.5485, 40.9768) (-30.6688, 40.7472) (-30.6688, 40.5996) knots 0 0 0 1 2 2 2
  spline S84 degree 2 poles (-30.6688, 40.5996) (-30.6688, 40.4247) (-30.3299, 40.1897) (-30.0457, 40.1788) knots 0 0 0 1 2 2 2
  line L215 (-30.0457, 40.1788) -> (-28.8158, 40.135)
  spline S85 degree 2 poles (-28.8158, 40.135) (-28.466, 40.1241) (-27.8702, 39.9656) (-27.4493, 39.665) (-27.2088, 39.2277) (-27.2088, 38.938) knots 0 0 0 1 2 3 4 4 4
  spline S86 degree 2 poles (-27.2088, 38.938) (-27.2088, 38.6264) (-27.4821, 38.0634) (-28.0451, 37.6371) (-28.9142, 37.3857) (-29.51, 37.3857) knots 0 0 0 1 2 3 4 4 4
  spline S87 degree 2 poles (-29.51, 37.3857) (-30.0785, 37.3857) (-30.8765, 37.566) (-31.3903, 37.8885) (-31.6253, 38.3313) (-31.6253, 38.5991) knots 0 0 0 1 2 3 4 4 4
  spline S88 degree 2 poles (-31.6253, 38.5991) (-31.6253, 38.9435) (-31.3083, 39.4573) (-30.9749, 39.6923) knots 0 0 0 1 2 2 2
  spline S89 degree 2 poles (-30.9749, 39.6923) (-31.1006, 39.747) (-31.2755, 39.9164) (-31.3903, 40.1186) (-31.445, 40.3427) (-31.445, 40.4521) knots 0 0 0 1 2 3 4 4 4
  spline S90 degree 2 poles (-31.445, 40.4521) (-31.445, 40.7527) (-31.1607, 41.2556) (-30.9639, 41.4797) knots 0 0 0 1 2 2 2
  spline S91 degree 2 poles (-30.9639, 41.4797) (-31.0514, 41.589) (-31.1881, 41.7967) (-31.2864, 42.0317) (-31.3356, 42.3105) (-31.3356, 42.4854) knots 0 0 0 1 2 3 4 4 4
  spline S92 degree 2 poles (-31.3356, 42.4854) (-31.3356, 42.8516) (-31.0678, 43.4529) (-30.5868, 43.8792) (-29.9145, 44.1197) (-29.5045, 44.1197) knots 0 0 0 1 2 3 4 4 4
  spline S93 degree 2 poles (-29.5045, 44.1197) (-29.3296, 44.1197) (-29.0126, 44.0705) (-28.8924, 44.0323) knots 0 0 0 1 2 2 2
  line L216 (-28.8924, 44.0323) -> (-27.1924, 44.0323)
  line L217 (-27.1924, 44.0323) -> (-27.1924, 43.3709)
  line L218 (-27.1924, 43.3709) -> (-27.9413, 43.3709)
  spline S94 degree 2 poles (-30.5157, 42.5073) (-30.5157, 42.2832) (-30.3682, 41.906) (-30.0949, 41.6436) (-29.7286, 41.5015) (-29.4991, 41.5015) knots 0 0 0 1 2 3 4 4 4
  spline S95 degree 2 poles (-29.4991, 41.5015) (-29.2586, 41.5015) (-28.8814, 41.6655) (-28.6245, 41.9443) (-28.4879, 42.3105) (-28.4879, 42.5073) knots 0 0 0 1 2 3 4 4 4
  spline S96 degree 2 poles (-28.4879, 42.5073) (-28.4879, 42.7259) (-28.6355, 43.103) (-28.9088, 43.3654) (-29.275, 43.5075) (-29.4991, 43.5075) knots 0 0 0 1 2 3 4 4 4
  spline S97 degree 2 poles (-29.4991, 43.5075) (-29.745, 43.5075) (-30.1222, 43.3381) (-30.3791, 43.0648) (-30.5157, 42.6986) (-30.5157, 42.5073) knots 0 0 0 1 2 3 4 4 4
  spline S98 degree 2 poles (-30.7617, 38.6702) (-30.7617, 38.3422) (-30.073, 38.0361) (-29.4553, 38.0361) knots 0 0 0 1 2 2 2
  spline S99 degree 2 poles (-29.4553, 38.0361) (-29.0673, 38.0361) (-28.5425, 38.1782) (-28.22, 38.4023) (-28.0779, 38.6975) (-28.0779, 38.8505) knots 0 0 0 1 2 3 4 4 4
  spline S100 degree 2 poles (-28.0779, 38.8505) (-28.0779, 39.1348) (-28.5425, 39.4081) (-29.0235, 39.4299) knots 0 0 0 1 2 2 2
  line L219 (-29.0235, 39.4299) -> (-30.2479, 39.4737)
  spline S101 degree 2 poles (-30.2479, 39.4737) (-30.401, 39.3698) (-30.6032, 39.173) (-30.7125, 38.9763) (-30.7617, 38.774) (-30.7617, 38.6702) knots 0 0 0 1 2 3 4 4 4
  line L220 (-38.2902, -42.2154) -> (-38.7617, -42.2154)
  line L221 (-38.7617, -42.2154) -> (-38.9804, -41.5252)
  line L222 (-38.9804, -41.5252) -> (-40.3069, -41.5252)
  line L223 (-40.3069, -41.5252) -> (-40.5285, -42.2154)
  line L224 (-40.5285, -42.2154) -> (-40.9744, -42.2154)
  line L225 (-40.9744, -42.2154) -> (-39.9234, -39.0454)
  line L226 (-39.9234, -39.0454) -> (-39.3298, -39.0454)
  line L227 (-39.3298, -39.0454) -> (-38.2902, -42.2154)
  line L228 (-39.1054, -41.1389) -> (-39.6422, -39.4403)
  line L229 (-39.6422, -39.4403) -> (-40.1848, -41.1389)
  line L230 (-40.1848, -41.1389) -> (-39.1054, -41.1389)
  line L231 (-36.1399, -42.2154) -> (-36.1399, -40.4657)
  spline S102 degree 2 poles (-36.1399, -40.4657) (-36.1399, -40.3521) (-36.1569, -40.2072) (-36.191, -40.122) (-36.2422, -40.0879) (-36.2819, -40.0879) knots 0 0 0 1 2 3 4 4 4
  spline S103 degree 2 poles (-36.2819, -40.0879) (-36.3274, -40.0879) (-36.4041, -40.1447) (-36.4921, -40.2782) (-36.5972, -40.4941) (-36.6711, -40.6503) knots 0 0 0 1 2 3 4 4 4
  line L232 (-36.6711, -40.6503) -> (-36.6711, -42.2154)
  line L233 (-36.6711, -42.2154) -> (-37.0943, -42.2154)
  line L234 (-37.0943, -42.2154) -> (-37.0943, -40.5111)
  spline S104 degree 2 poles (-37.0943, -40.5111) (-37.0943, -40.3776) (-37.1114, -40.2129) (-37.1454, -40.122) (-37.1994, -40.0879) (-37.2392, -40.0879) knots 0 0 0 1 2 3 4 4 4
  spline S105 degree 2 poles (-37.2392, -40.0879) (-37.2789, -40.0879) (-37.3528, -40.1362) (-37.4409, -40.2612) (-37.5516, -40.4799) (-37.6255, -40.6503) knots 0 0 0 1 2 3 4 4 4
  line L235 (-37.6255, -40.6503) -> (-37.6255, -42.2154)
  line L236 (-37.6255, -42.2154) -> (-38.0487, -42.2154)
  line L237 (-38.0487, -42.2154) -> (-38.0487, -39.7811)
  line L238 (-38.0487, -39.7811) -> (-37.6965, -39.7811)
  line L239 (-37.6965, -39.7811) -> (-37.6766, -40.2441)
  spline S106 degree 2 poles (-37.6766, -40.2441) (-37.6113, -40.105) (-37.492, -39.9118) (-37.367, -39.7925) (-37.2221, -39.7357) (-37.1369, -39.7357) knots 0 0 0 1 2 3 4 4 4
  spline S107 degree 2 poles (-37.1369, -39.7357) (-36.9381, -39.7357) (-36.7336, -39.9942) (-36.7336, -40.264) knots 0 0 0 1 2 2 2
  spline S108 degree 2 poles (-36.7336, -40.264) (-36.6768, -40.1362) (-36.5631, -39.9402) (-36.4353, -39.8067) (-36.2791, -39.7357) (-36.1768, -39.7357) knots 0 0 0 1 2 3 4 4 4
  spline S109 degree 2 poles (-36.1768, -39.7357) (-35.7167, -39.7357) (-35.7167, -40.443) knots 0 0 0 1 1 1
  line L240 (-35.7167, -40.443) -> (-35.7167, -42.2154)
  line L241 (-35.7167, -42.2154) -> (-36.1399, -42.2154)
  spline S110 degree 2 poles (-33.0665, -40.9543) (-33.0665, -41.2781) (-33.2483, -41.7638) (-33.5664, -42.0848) (-34.0038, -42.2439) (-34.2566, -42.2439) knots 0 0 0 1 2 3 4 4 4
  spline S111 degree 2 poles (-34.2566, -42.2439) (-34.3731, -42.2439) (-34.6032, -42.2211) (-34.7225, -42.1899) knots 0 0 0 1 2 2 2
  line L242 (-34.7225, -42.1899) -> (-34.7225, -43.2096)
  line L243 (-34.7225, -43.2096) -> (-35.1457, -43.2096)
  line L244 (-35.1457, -43.2096) -> (-35.1457, -39.7811)
  line L245 (-35.1457, -39.7811) -> (-34.7679, -39.7811)
  line L246 (-34.7679, -39.7811) -> (-34.7424, -40.1873)
  spline S112 degree 2 poles (-34.7424, -40.1873) (-34.5606, -39.9374) (-34.1487, -39.7357) (-33.9101, -39.7357) knots 0 0 0 1 2 2 2
  spline S113 degree 2 poles (-33.9101, -39.7357) (-33.6999, -39.7357) (-33.3875, -39.909) (-33.1716, -40.2271) (-33.0665, -40.6759) (-33.0665, -40.9543) knots 0 0 0 1 2 3 4 4 4
  spline S114 degree 2 poles (-33.4982, -40.9741) (-33.4982, -40.781) (-33.555, -40.4629) (-33.6743, -40.2328) (-33.8647, -40.105) (-33.9953, -40.105) knots 0 0 0 1 2 3 4 4 4
  spline S115 degree 2 poles (-33.9953, -40.105) (-34.0749, -40.105) (-34.2396, -40.1561) (-34.4157, -40.2754) (-34.6117, -40.4714) (-34.7225, -40.6162) knots 0 0 0 1 2 3 4 4 4
  line L247 (-34.7225, -40.6162) -> (-34.7225, -41.7979)
  spline S116 degree 2 poles (-34.7225, -41.7979) (-34.606, -41.8462) (-34.3504, -41.903) (-34.2254, -41.903) knots 0 0 0 1 2 2 2
  spline S117 degree 2 poles (-34.2254, -41.903) (-33.8845, -41.903) (-33.4982, -41.44) (-33.4982, -40.9741) knots 0 0 0 1 2 2 2
  line L248 (-30.6748, -42.2154) -> (-30.6748, -40.4657)
  spline S118 degree 2 poles (-30.6748, -40.4657) (-30.6748, -40.3521) (-30.6918, -40.2072) (-30.7259, -40.122) (-30.777, -40.0879) (-30.8168, -40.0879) knots 0 0 0 1 2 3 4 4 4
  spline S119 degree 2 poles (-30.8168, -40.0879) (-30.8622, -40.0879) (-30.9389, -40.1447) (-31.027, -40.2782) (-31.1321, -40.4941) (-31.2059, -40.6503) knots 0 0 0 1 2 3 4 4 4
  line L249 (-31.2059, -40.6503) -> (-31.2059, -42.2154)
  line L250 (-31.2059, -42.2154) -> (-31.6292, -42.2154)
  line L251 (-31.6292, -42.2154) -> (-31.6292, -40.5111)
  spline S120 degree 2 poles (-31.6292, -40.5111) (-31.6292, -40.3776) (-31.6462, -40.2129) (-31.6803, -40.122) (-31.7343, -40.0879) (-31.7741, -40.0879) knots 0 0 0 1 2 3 4 4 4
  spline S121 degree 2 poles (-31.7741, -40.0879) (-31.8138, -40.0879) (-31.8877, -40.1362) (-31.9757, -40.2612) (-32.0865, -40.4799) (-32.1604, -40.6503) knots 0 0 0 1 2 3 4 4 4
  line L252 (-32.1604, -40.6503) -> (-32.1604, -42.2154)
  line L253 (-32.1604, -42.2154) -> (-32.5836, -42.2154)
  line L254 (-32.5836, -42.2154) -> (-32.5836, -39.7811)
  line L255 (-32.5836, -39.7811) -> (-32.2314, -39.7811)
  line L256 (-32.2314, -39.7811) -> (-32.2115, -40.2441)
  spline S122 degree 2 poles (-32.2115, -40.2441) (-32.1462, -40.105) (-32.0269, -39.9118) (-31.9019, -39.7925) (-31.757, -39.7357) (-31.6718, -39.7357) knots 0 0 0 1 2 3 4 4 4
  spline S123 degree 2 poles (-31.6718, -39.7357) (-31.473, -39.7357) (-31.2684, -39.9942) (-31.2684, -40.264) knots 0 0 0 1 2 2 2
  spline S124 degree 2 poles (-31.2684, -40.264) (-31.2116, -40.1362) (-31.098, -39.9402) (-30.9702, -39.8067) (-30.814, -39.7357) (-30.7117, -39.7357) knots 0 0 0 1 2 3 4 4 4
  spline S125 degree 2 poles (-30.7117, -39.7357) (-30.2515, -39.7357) (-30.2515, -40.443) knots 0 0 0 1 1 1
  line L257 (-30.2515, -40.443) -> (-30.2515, -42.2154)
  line L258 (-30.2515, -42.2154) -> (-30.6748, -42.2154)
  spline S126 degree 2 poles (-27.6241, -40.8691) (-27.6241, -40.9571) (-27.6298, -41.0792) (-27.6326, -41.1332) knots 0 0 0 1 2 2 2
  line L259 (-27.6326, -41.1332) -> (-29.3454, -41.1332)
  spline S127 degree 2 poles (-29.3454, -41.1332) (-29.3454, -41.5053) (-28.9279, -41.9058) (-28.533, -41.9058) knots 0 0 0 1 2 2 2
  spline S128 degree 2 poles (-28.533, -41.9058) (-28.4279, -41.9058) (-28.2149, -41.8888) (-28.0132, -41.8604) (-27.8314, -41.8235) (-27.7547, -41.8007) knots 0 0 0 1 2 3 4 4 4
  line L260 (-27.7547, -41.8007) -> (-27.7547, -42.1473)
  spline S129 degree 2 poles (-27.7547, -42.1473) (-27.928, -42.1956) (-28.3626, -42.2581) (-28.5955, -42.2581) knots 0 0 0 1 2 2 2
  spline S130 degree 2 poles (-28.5955, -42.2581) (-28.908, -42.2581) (-29.3596, -42.0876) (-29.6465, -41.7666) (-29.7857, -41.298) (-29.7857, -41.0026) knots 0 0 0 1 2 3 4 4 4
  spline S131 degree 2 poles (-29.7857, -41.0026) (-29.7857, -40.7441) (-29.638, -40.2867) (-29.3539, -39.9402) (-28.9421, -39.7357) (-28.6807, -39.7357) knots 0 0 0 1 2 3 4 4 4
  spline S132 degree 2 poles (-28.6807, -39.7357) (-28.4251, -39.7357) (-28.0303, -39.8948) (-27.7633, -40.1902) (-27.6241, -40.6077) (-27.6241, -40.8691) knots 0 0 0 1 2 3 4 4 4
  spline S133 degree 2 poles (-28.0644, -40.8094) (-28.0558, -40.6475) (-28.1354, -40.3776) (-28.2973, -40.1816) (-28.5387, -40.0737) (-28.7006, -40.0737) knots 0 0 0 1 2 3 4 4 4
  spline S134 degree 2 poles (-28.7006, -40.0737) (-28.837, -40.0737) (-29.0671, -40.1816) (-29.2318, -40.3748) (-29.3341, -40.6475) (-29.3454, -40.8094) knots 0 0 0 1 2 3 4 4 4
  line L261 (-29.3454, -40.8094) -> (-28.0644, -40.8094)
  spline S135 degree 2 poles (-24.9853, -42.1814) (-25.1273, -42.2183) (-25.4341, -42.2495) (-25.5931, -42.2495) knots 0 0 0 1 2 2 2
  spline S136 degree 2 poles (-25.5931, -42.2495) (-26.0504, -42.2495) (-26.5021, -41.8348) (-26.5021, -41.4059) knots 0 0 0 1 2 2 2
  line L262 (-26.5021, -41.4059) -> (-26.5021, -40.1362)
  line L263 (-26.5021, -40.1362) -> (-27.1838, -40.1362)
  line L264 (-27.1838, -40.1362) -> (-27.1838, -39.7811)
  line L265 (-27.1838, -39.7811) -> (-26.5021, -39.7811)
  line L266 (-26.5021, -39.7811) -> (-26.5021, -39.1108)
  line L267 (-26.5021, -39.1108) -> (-26.0788, -39.0028)
  line L268 (-26.0788, -39.0028) -> (-26.0788, -39.7811)
  line L269 (-26.0788, -39.7811) -> (-24.9853, -39.7811)
  line L270 (-24.9853, -39.7811) -> (-24.9853, -40.1362)
  line L271 (-24.9853, -40.1362) -> (-26.0788, -40.1362)
  line L272 (-26.0788, -40.1362) -> (-26.0788, -41.3718)
  spline S137 degree 2 poles (-26.0788, -41.3718) (-26.0788, -41.6331) (-25.8005, -41.8916) (-25.5278, -41.8916) knots 0 0 0 1 2 2 2
  spline S138 degree 2 poles (-25.5278, -41.8916) (-25.4113, -41.8916) (-25.1358, -41.8547) (-24.9853, -41.8178) knots 0 0 0 1 2 2 2
  line L273 (-24.9853, -41.8178) -> (-24.9853, -42.1814)
  spline S139 degree 2 poles (-22.159, -40.8691) (-22.159, -40.9571) (-22.1646, -41.0792) (-22.1675, -41.1332) knots 0 0 0 1 2 2 2
  line L274 (-22.1675, -41.1332) -> (-23.8803, -41.1332)
  spline S140 degree 2 poles (-23.8803, -41.1332) (-23.8803, -41.5053) (-23.4627, -41.9058) (-23.0679, -41.9058) knots 0 0 0 1 2 2 2
  spline S141 degree 2 poles (-23.0679, -41.9058) (-22.9628, -41.9058) (-22.7498, -41.8888) (-22.5481, -41.8604) (-22.3663, -41.8235) (-22.2896, -41.8007) knots 0 0 0 1 2 3 4 4 4
  line L275 (-22.2896, -41.8007) -> (-22.2896, -42.1473)
  spline S142 degree 2 poles (-22.2896, -42.1473) (-22.4629, -42.1956) (-22.8975, -42.2581) (-23.1304, -42.2581) knots 0 0 0 1 2 2 2
  spline S143 degree 2 poles (-23.1304, -42.2581) (-23.4429, -42.2581) (-23.8945, -42.0876) (-24.1814, -41.7666) (-24.3206, -41.298) (-24.3206, -41.0026) knots 0 0 0 1 2 3 4 4 4
  spline S144 degree 2 poles (-24.3206, -41.0026) (-24.3206, -40.7441) (-24.1729, -40.2867) (-23.8888, -39.9402) (-23.4769, -39.7357) (-23.2156, -39.7357) knots 0 0 0 1 2 3 4 4 4
  spline S145 degree 2 poles (-23.2156, -39.7357) (-22.96, -39.7357) (-22.5651, -39.8948) (-22.2981, -40.1902) (-22.159, -40.6077) (-22.159, -40.8691) knots 0 0 0 1 2 3 4 4 4
  spline S146 degree 2 poles (-22.5992, -40.8094) (-22.5907, -40.6475) (-22.6702, -40.3776) (-22.8322, -40.1816) (-23.0736, -40.0737) (-23.2355, -40.0737) knots 0 0 0 1 2 3 4 4 4
  spline S147 degree 2 poles (-23.2355, -40.0737) (-23.3718, -40.0737) (-23.6019, -40.1816) (-23.7667, -40.3748) (-23.8689, -40.6475) (-23.8803, -40.8094) knots 0 0 0 1 2 3 4 4 4
  line L276 (-23.8803, -40.8094) -> (-22.5992, -40.8094)
  line L277 (-21.3835, -39.7811) -> (-20.9972, -39.7811)
  line L278 (-20.9972, -39.7811) -> (-20.9858, -40.2299)
  spline S148 degree 2 poles (-20.9858, -40.2299) (-20.7699, -39.9686) (-20.3524, -39.7357) (-20.1365, -39.7357) knots 0 0 0 1 2 2 2
  spline S149 degree 2 poles (-20.1365, -39.7357) (-19.7587, -39.7357) (-19.3696, -40.2271) (-19.3838, -40.71) knots 0 0 0 1 2 2 2
  line L279 (-19.3838, -40.71) -> (-19.8099, -40.71)
  spline S150 degree 2 poles (-19.8099, -40.71) (-19.8013, -40.389) (-20.003, -40.0993) (-20.199, -40.0993) knots 0 0 0 1 2 2 2
  spline S151 degree 2 poles (-20.199, -40.0993) (-20.2842, -40.0993) (-20.4547, -40.1589) (-20.6364, -40.2953) (-20.841, -40.5026) (-20.9574, -40.6532) knots 0 0 0 1 2 3 4 4 4
  line L280 (-20.9574, -40.6532) -> (-20.9574, -42.2154)
  line L281 (-20.9574, -42.2154) -> (-21.3835, -42.2154)
  line L282 (-21.3835, -42.2154) -> (-21.3835, -39.7811)
  spline S152 degree 2 poles (-13.8903, -40.6304) (-13.8903, -40.994) (-14.0351, -41.5934) (-14.3305, -42.0223) (-14.7708, -42.2581) (-15.0662, -42.2581) knots 0 0 0 1 2 3 4 4 4
  spline S153 degree 2 poles (-15.0662, -42.2581) (-15.3219, -42.2581) (-15.7366, -42.0677) (-16.0348, -41.6672) (-16.1939, -41.0537) (-16.1939, -40.6304) knots 0 0 0 1 2 3 4 4 4
  spline S154 degree 2 poles (-16.1939, -40.6304) (-16.1939, -40.2669) (-16.0462, -39.6647) (-15.7536, -39.2358) (-15.3105, -39) (-15.0179, -39) knots 0 0 0 1 2 3 4 4 4
  spline S155 degree 2 poles (-15.0179, -39) (-14.7623, -39) (-14.3447, -39.1903) (-14.0493, -39.5908) (-13.8903, -40.2072) (-13.8903, -40.6304) knots 0 0 0 1 2 3 4 4 4
  spline S156 degree 2 poles (-14.3163, -40.6447) (-14.3163, -40.5623) (-14.3277, -40.4004) (-14.3362, -40.3237) knots 0 0 0 1 2 2 2
  line L283 (-14.3362, -40.3237) -> (-15.6769, -41.3178)
  spline S157 degree 2 poles (-15.6769, -41.3178) (-15.6428, -41.4457) (-15.5292, -41.6587) (-15.373, -41.8121) (-15.1713, -41.8973) (-15.0407, -41.8973) knots 0 0 0 1 2 3 4 4 4
  spline S158 degree 2 poles (-15.0407, -41.8973) (-14.8759, -41.8973) (-14.6089, -41.7382) (-14.4186, -41.4201) (-14.3163, -40.9514) (-14.3163, -40.6447) knots 0 0 0 1 2 3 4 4 4
  spline S159 degree 2 poles (-15.7678, -40.6162) (-15.7678, -40.6901) (-15.765, -40.8406) (-15.7593, -40.9117) knots 0 0 0 1 2 2 2
  line L284 (-15.7593, -40.9117) -> (-14.4157, -39.9203)
  spline S160 degree 2 poles (-14.4157, -39.9203) (-14.4527, -39.7953) (-14.5634, -39.5908) (-14.7197, -39.4431) (-14.9185, -39.3607) (-15.0407, -39.3607) knots 0 0 0 1 2 3 4 4 4
  spline S161 degree 2 poles (-15.0407, -39.3607) (-15.2082, -39.3607) (-15.4753, -39.5198) (-15.6656, -39.8379) (-15.7678, -40.3066) (-15.7678, -40.6162) knots 0 0 0 1 2 3 4 4 4
  line L285 (-8.8512, -41.0934) -> (-10.3027, -41.0934)
  line L286 (-10.3027, -41.0934) -> (-10.3027, -40.6958)
  line L287 (-10.3027, -40.6958) -> (-8.8512, -40.6958)
  line L288 (-8.8512, -40.6958) -> (-8.8512, -41.0934)
  line L289 (-3.031, -42.2154) -> (-5.1188, -42.2154)
  line L290 (-5.1188, -42.2154) -> (-5.1188, -41.8377)
  line L291 (-5.1188, -41.8377) -> (-4.3007, -41.0224)
  spline S162 degree 2 poles (-4.3007, -41.0224) (-4.099, -40.8236) (-3.8462, -40.531) (-3.7071, -40.2896) (-3.6588, -40.0766) (-3.6588, -39.9544) knots 0 0 0 1 2 3 4 4 4
  spline S163 degree 2 poles (-3.6588, -39.9544) (-3.6588, -39.8379) (-3.7213, -39.6278) (-3.8519, -39.4658) (-4.0621, -39.3749) (-4.207, -39.3749) knots 0 0 0 1 2 3 4 4 4
  spline S164 degree 2 poles (-4.207, -39.3749) (-4.4087, -39.3749) (-4.7382, -39.5539) (-4.8745, -39.6988) knots 0 0 0 1 2 2 2